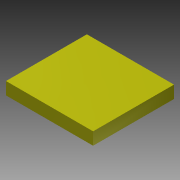
# Autodesk Inventor part: Bench_Part1
Saved by Autodesk Inventor 2015 SP2 (Build 190223200, 223)
## iProperties
Created: 2017-05-28
Part Number: Bench_Part1
Material: Stainless Steel
Document SubType Name: Modeling
Designer: MehariK
Density: 8 g/cm^3
Appearance: Yellow
Author: MehariK
Autodesk Inventor part; units mm, degrees
ref_plane "YZ Plane" through (0, 0, 0) normal (1, 0, 0) x (0, 1, 0)
ref_plane "XZ Plane" through (0, 0, 0) normal (0, 1, 0) x (-1, 0, 0)
ref_plane "XY Plane" through (0, 0, 0) normal (0, 0, 1) x (1, 0, 0)
sketch "Sketch1" plane through (0, 0, 0) normal (0, 1, 0) x (-1, 0, 0)
  line L0 (0, 0) -> (-700, 0)
  line L1 (-700, 0) -> (-700, -100)
  line L2 (-700, -100) -> (0, -100)
  line L3 (0, -100) -> (0, 0)
  dimension "d0" = 700
  dimension "d1" = 100
  constraints: 8 end point, 2 parallel, 1 horizontal, 1 perpendicular
  measures "d0" distance of L2.end L1.end
  measures "d1" distance of L0.end L1.end
extrude "Extrusion1" add sketch "Sketch1" along normal blind 650
body "Solid1"
